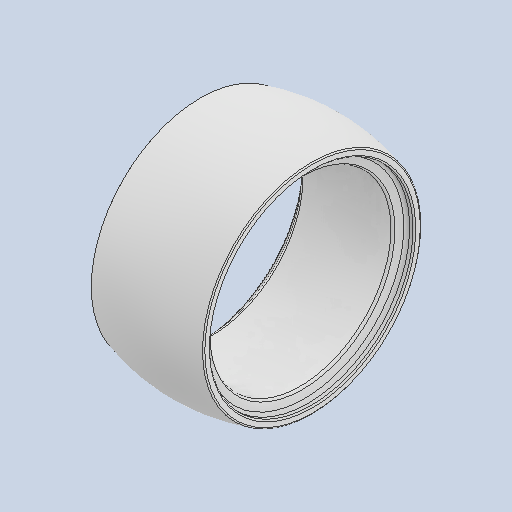
# Autodesk Inventor part: ToePalm
Saved by Autodesk Inventor 2022.2 (Build 262287000, 287)
## iProperties
Created: 2021-12-28
Part Number: ToePalm
Material: Generic
Document SubType Name: Modeling
Designer: Jochen
Density: 1 g/cm^3
Appearance: Default
Author: Jochen
Autodesk Inventor part; units mm, degrees
ref_plane "YZ Plane" through (0, 0, 0) normal (1, 0, 0) x (0, 1, 0)
ref_plane "XZ Plane" through (0, 0, 0) normal (0, 1, 0) x (-1, 0, 0)
ref_plane "XY Plane" through (0, 0, 0) normal (0, 0, 1) x (1, 0, 0)
derived "Toe.ipt"
sketch "ToeSketch" plane through (0, 0, 0) normal (0, 0, 1) x (1, 0, 0)
  line L0 (-11.666, 0) -> (11.666, 0) construction
  line L1 (0, -16.1502) -> (0, 19.9967) construction
  line L2 (-8.25, 12.3131) -> (-8.25, 11.6707)
  line L3 (8.25, 12.3131) -> (8.25, 11.6707)
  line L4 (0.75, 0.625) -> (0.75, 10.5)
  line L5 (0.75, 0.625) -> (-0.75, 0.625)
  line L6 (-0.75, 0.625) -> (-0.75, 10.5)
  line L7 (-7.85, 11.2707) -> (-7.1375, 11.2707)
  arc A0 (-2.8705, 11.5882) -> (-6.8566, 11.3859) centre (-4.75, 9.25) ccw
  arc A1 (6.8566, 11.3859) -> (2.8705, 11.5882) centre (4.75, 9.25) ccw
  line L8 (7.1375, 11.2707) -> (7.85, 11.2707)
  line L9 (-2.6199, 11.5) -> (-1.75, 11.5)
  line L10 (1.75, 11.5) -> (2.6199, 11.5)
  arc A2 (7.85, 11.2707) -> (8.25, 11.6707) centre (7.85, 11.6707) ccw
  arc A3 (8.25, 12.3131) -> (7.9777, 12.6922) centre (7.85, 12.3131) ccw
  arc A4 (-6.3927, 13.1684) -> (-8.25, 12.3131) centre (-7.3214, 12.7408) ccw
  arc A5 (-8.25, 11.6707) -> (-7.85, 11.2707) centre (-7.85, 11.6707) ccw
  arc A6 (-7.1375, 11.2707) -> (-6.8566, 11.3859) centre (-7.1375, 11.6707) ccw
  arc A7 (6.8566, 11.3859) -> (7.1375, 11.2707) centre (7.1375, 11.6707) ccw
  arc A8 (6.3927, 13.1684) -> (-6.3927, 13.1684) centre (0, -10.9864) ccw
  arc A9 (-2.8705, 11.5882) -> (-2.6199, 11.5) centre (-2.6199, 11.9) ccw
  arc A10 (2.6199, 11.5) -> (2.8705, 11.5882) centre (2.6199, 11.9) ccw
  arc A11 (-0.75, 10.5) -> (-1.75, 11.5) centre (-1.75, 10.5) ccw
  arc A12 (1.75, 11.5) -> (0.75, 10.5) centre (1.75, 10.5) ccw
  circle A13 centre (-4.75, 9.25) radius 3 construction
  circle A14 centre (4.75, 9.25) radius 3 construction
  line L11 (5.4355, 12.1706) -> (5.7098, 13.3389) construction
  line L12 (7.9777, 12.6922) -> (7.4988, 11.2707) construction
  line L13 (-7.2, 11.2707) -> (-7.2, 10.6)
  line L14 (-6.4, 9.8) -> (6.4, 9.8)
  line L15 (7.2, 10.6) -> (7.2, 11.2707)
  arc A15 (6.4, 9.8) -> (7.2, 10.6) centre (6.4, 10.6) ccw
  arc A16 (-7.2, 10.6) -> (-6.4, 9.8) centre (-6.4, 10.6) ccw
  line L16 (8.25, 12.3131) -> (8.25, 14.35)
  line L17 (7.85, 14.75) -> (7.55, 14.75)
  line L18 (7.0882, 14.35) -> (7.0882, 14.1857)
  line L19 (-8.25, 12.3131) -> (-8.25, 14.35)
  line L20 (-7.85, 14.75) -> (-7.55, 14.75)
  arc A17 (8.25, 14.35) -> (7.85, 14.75) centre (7.85, 14.35) ccw
  arc A18 (7.55, 14.75) -> (7.165, 14.4584) centre (7.55, 14.35) ccw
  arc A19 (-7.165, 14.4584) -> (-7.55, 14.75) centre (-7.55, 14.35) ccw
  arc A20 (-7.85, 14.75) -> (-8.25, 14.35) centre (-7.85, 14.35) ccw
  arc A21 (-6.8801, 13.4466) -> (-6.3927, 13.1684) centre (-6.495, 13.5551) ccw
  arc A22 (6.3927, 13.1684) -> (6.8801, 13.4466) centre (6.495, 13.5551) ccw
  line L21 (-7.165, 14.4584) -> (-6.8801, 13.4466)
  line L22 (6.8801, 13.4466) -> (7.165, 14.4584)
  point P0 (0, 0)
  point P1 (-8.25, 10.6859)
  point P2 (8.25, 10.6859)
  point P3 (8.25, 11.2707)
  point P4 (-6.9674, 11.2707)
  point P5 (-2.7657, 11.5)
  point P6 (2.7657, 11.5)
  point P7 (0, 14)
  point P8 (6.9674, 11.2707)
  point P9 (0.75, 11.5)
  point P10 (-7.2, 9.8)
  point P11 (7.2, 9.8)
sketch "Sketch2" plane through (0, 0, 0) normal (0, 0, 1) x (1, 0, 0)
  line L0 (0, -16.6036) -> (0, 22.7173) construction
  line L1 (-12.0797, 0) -> (11.7349, 0) construction
  arc A0 (8.1077, 15.9043) -> (-8.1077, 15.9043) centre (0, -10.9864) ccw
  arc A1 (7.9777, 12.6922) -> (-6.3927, 13.1684) centre (0, -10.9864) ccw construction
  line L2 (-8.25, 12.3131) -> (-8.25, 11.6707) construction
  arc A2 (8.25, 12.3131) -> (7.9777, 12.6922) centre (7.85, 12.3131) ccw construction
  line L3 (8.25, 12.3131) -> (8.25, 11.6707) construction
  arc A3 (6.4183, 13.2651) -> (-6.4183, 13.2651) centre (0, -10.9864) ccw
  line L4 (-7.85, 11.2707) -> (-7.1375, 11.2707) construction
  arc A4 (-8.25, 11.6707) -> (-7.85, 11.2707) centre (-7.85, 11.6707) ccw construction
  line L5 (7.1375, 11.2707) -> (7.85, 11.2707) construction
  arc A5 (7.85, 11.2707) -> (8.25, 11.6707) centre (7.85, 11.6707) ccw construction
  arc A6 (-6.7838, 13.4738) -> (-6.4183, 13.2651) centre (-6.495, 13.5551) ccw
  arc A7 (6.4183, 13.2651) -> (6.7838, 13.4738) centre (6.495, 13.5551) ccw
  line L6 (7.55, 14.85) -> (8.05, 14.85)
  arc A8 (8.05, 14.85) -> (8.25, 15.05) centre (8.05, 15.05) ccw
  line L7 (-7.55, 14.85) -> (-8.05, 14.85)
  arc A9 (-8.25, 15.05) -> (-8.05, 14.85) centre (-8.05, 15.05) ccw
  line L8 (8.25, 14.35) -> (8.25, 15.05) construction
  line L9 (8.25, 12.3131) -> (8.25, 14.35) construction
  arc A10 (-7.0687, 14.4855) -> (-7.55, 14.85) centre (-7.55, 14.35) ccw
  line L10 (-7.0687, 14.4855) -> (-6.7838, 13.4738)
  line L11 (-7.165, 14.4584) -> (-6.8801, 13.4466) construction
  line L12 (6.7838, 13.4738) -> (7.0687, 14.4855)
  arc A11 (7.55, 14.85) -> (7.0687, 14.4855) centre (7.55, 14.35) ccw
  line L13 (8.25, 15.05) -> (8.25, 15.7128)
  arc A12 (8.25, 15.7128) -> (8.1077, 15.9043) centre (8.05, 15.7128) ccw
  line L14 (-8.25, 15.05) -> (-8.25, 15.7128)
  arc A13 (-8.1077, 15.9043) -> (-8.25, 15.7128) centre (-8.05, 15.7128) ccw
  point P0 (0, 0)
  point P1 (0, 17.1)
  point P2 (7.55, 14.35)
  dimension "d3" = 3
  dimension "d6" = 0.1
  dimension "d19" = 0.2
  constraints: 21 point on circle, 14 end point, 14 tangent, 10 centre point, 2 coincident, 2 collinear, 2 concentric, 2 horizontal, 2 vertical, 1 equal radius, 1 parallel, 6 other
  measures "d3" radial gap between concentric circles of A0 A3
  measures "d6" radial gap between concentric circles of A3 A1
  measures "d19" radius of A8
revolve "Revolution1" add sketch "Sketch2" angle 360 about axis through (-10, 0, 0) along (1, 0, 0)
body "Solid1"
